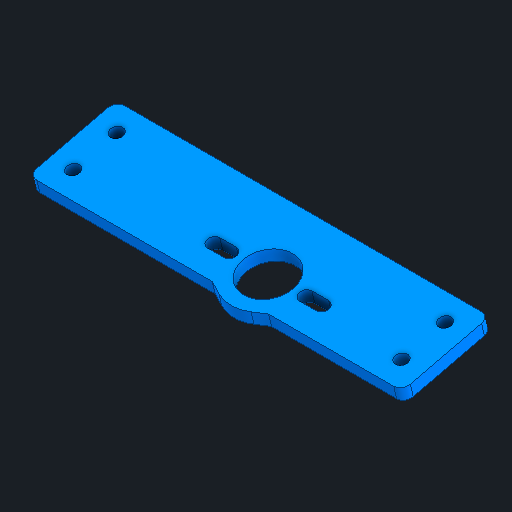
# Autodesk Inventor part: motor_mount_plate
Saved by Autodesk Inventor 2024 (Build 280153000, 153)
## iProperties
Created: 2022-03-30
Part Number: motor_mount_plate
Material: Generic
Document SubType Name: Modeling
Designer: kardo
Density: 1 g/cm^3
Appearance: Blue Plastic
Mass: 3.74158 g
Surface Area: 43.0769 cm^2
Volume: 3.74158 cm^3
Author: kardo
Autodesk Inventor part; units mm, degrees
ref_plane "YZ Plane" through (0, 0, 0) normal (1, 0, 0) x (0, 1, 0)
ref_plane "XZ Plane" through (0, 0, 0) normal (0, 1, 0) x (-1, 0, 0)
ref_plane "XY Plane" through (0, 0, 0) normal (0, 0, 1) x (1, 0, 0)
derived "stencil_frame.ipt"
sketch "sk_cowl_joint_locations" plane through (54.6, 0, 0) normal (1, 0, 0) x (0, 1, 0)
  line L0 (-345, 16.32) -> (-262.2001, 18.586) construction
  arc A0 (-262.2001, 18.586) -> (-241.5001, 19.2432) centre (-326.8578, 2381.2399) ccw construction
  line L1 (-241.5001, 19.2432) -> (11.22, 28.376) construction
  arc A1 (36.465, 28.832) -> (11.22, 28.376) centre (36.465, -670.197) ccw construction
  line L2 (36.465, 28.832) -> (112.2, 28.832) construction
  line L3 (94.8, 29.632) -> (36.465, 29.632) construction
  arc A2 (36.465, 29.632) -> (11.1911, 29.1755) centre (36.465, -670.197) ccw construction
  line L4 (11.1911, 29.1755) -> (-241.529, 20.0427) construction
  arc A3 (-262.222, 19.3857) -> (-241.529, 20.0427) centre (-326.8578, 2381.2399) ccw construction
  line L5 (-262.222, 19.3857) -> (-345, 17.1203) construction
  line L6 (-230.0001, 3089.1136) -> (-230.0001, -1866.0023) construction
  line L7 (-114.9999, 3089.1136) -> (-114.9999, -1866.0023) construction
  line L8 (-345, 3089.1136) -> (-345, -1866.0023) construction
  line L9 (0, 3089.1136) -> (0, -1866.0023) construction
  line L10 (-230.0001, 44.8681) -> (-230.0001, 20.4593) construction
  line L11 (-114.9999, 49.7658) -> (-114.9999, 24.6152) construction
  line L12 (-345, 17.1203) -> (-345, 17.1203)
  line L13 (-345, 17.1203) -> (-345, 36.7228) construction
  line L14 (-850.7464, 3011.9134) -> (325.2296, -1886.3794) construction
  line L15 (-344.7454, 36.7228) -> (-345, 39.712) construction
  line L16 (0, 51.4) -> (0, 28.7711) construction
  line L17 (-144.5331, 44.6212) -> (-139.5174, 23.7292) construction
  line L18 (-134.9371, 30.3529) -> (-140.7713, 28.9522) construction
  line L19 (-137.4449, 40.7989) -> (-143.2792, 39.3982) construction
  line L20 (-144.5331, 44.6212) -> (-138.6989, 46.0219) construction
  line L21 (-139.5174, 23.7292) -> (-133.6831, 25.1299) construction
  line L22 (-138.6989, 46.0219) -> (-138.9044, 52.0184) construction
  spline S0 degree 2 poles (-345, 39.712) (-172.656, 54.3934) (0, 54.4) knots 0 0 0 1 1 1
  spline S1 degree 3 poles (0, 54.4) (37.026, 54.4) (80.784, 47.9917) (112.2, 37.536) knots 1 1 1 1 2 2 2 2
  spline S2 degree 3 poles (111.2526, 34.6895) (106.0906, 36.4075) (96.4401, 39.2282) (84.5011, 42.0313) (75.2591, 43.9395) (68.9709, 45.1125) (60.9945, 46.449) (54.5373, 47.4124) (46.413, 48.4791) (39.8882, 49.2203) (31.7426, 50.0013) (25.2514, 50.5076) (17.2112, 50.9875) (9.2661, 51.3118) (3.0567, 51.4) (0, 51.4) knots 1 1 1 1 1.166667 1.291667 1.333333 1.416667 1.458333 1.541667 1.583333 1.666667 1.708333 1.791667 1.833333 1.916667 2 2 2 2
  spline S3 degree 3 poles (0, 51.4) (-19.1698, 51.3993) (-52.712, 51.1604) (-91.0357, 50.4121) (-119.7742, 49.6473) (-138.931, 49.0355) (-162.8744, 48.1436) (-182.0269, 47.3282) (-205.9648, 46.1816) (-225.113, 45.1626) (-249.0455, 43.7615) (-268.1894, 42.5387) (-292.1166, 40.883) (-316.041, 39.1) (-335.1777, 37.5379) (-344.7454, 36.7228) knots 0 0 0 0 0.166667 0.291667 0.333333 0.416667 0.458333 0.541666 0.583333 0.666666 0.708333 0.791666 0.833333 0.916666 1 1 1 1
  point P0 (0, 0)
  point P1 (-345, 26.9216)
  point P2 (-230.0001, 32.6637)
  point P3 (-114.9999, 37.1905)
  point P4 (0, 40.0855)
  point P5 (0, 40.0855)
ref_plane "plane_motor_mount" through (0, -127.65, 0) normal (0, 0.9723699, 0.2334454) x (-1, 0, 0)
ref_plane "plane_symmetry" through (0, 0, 0) normal (1, 0, 0) x (0, 1, 0)
sketch "sk_drivetrain_profile" plane through (6, 0, 0) normal (1, 0, 0) x (0, 1, 0)
  line L0 (-529.1844, 0) -> (410.1064, 0) construction
  line L1 (-345, 3089.1136) -> (-345, -1866.0023) construction
  line L2 (0, 3089.1136) -> (0, -1866.0023) construction
  line L3 (-140.3859, 53.0487) -> (-133.8494, 25.8223)
  line L4 (-377, 0) -> (-313.1973, 5.0214)
  line L5 (-137.1176, 39.4355) -> (-233.3061, 16.3427)
  line L6 (-296.4782, 6.3372) -> (-264.4984, 8.8541) construction
  line L7 (-264.4984, 8.8541) -> (-233.3061, 16.3427) construction
  line L8 (-133.8494, 25.8223) -> (-133.8494, 20.8223) construction
  line L9 (-313.1973, 5.0214) -> (-296.4782, 6.3372)
  line L10 (-850.7464, 3011.9134) -> (325.2296, -1886.3794) construction
  line L11 (-233.9547, 19.044) -> (-137.7662, 42.1369) construction
  line L12 (-136.4691, 36.7341) -> (-232.6576, 13.6413) construction
  line L13 (-233.9547, 19.044) -> (-232.6576, 13.6413) construction
  spline S0 degree 2 poles (-296.4782, 6.3372) (-264.4984, 8.8541) (-233.3061, 16.3427) knots 1 1 1 2 2 2
  line L14 (0, 21.3303) -> (-241.5001, 18.9703) construction
  line L15 (-55.7851, 21.5852) -> (-309.9218, 19.1017) construction
  point P0 (0, 0)
  point P1 (-221.5492, 19.1653)
  point P2 (-209.1437, 19.2865)
  point P3 (-205.6699, 20.1205)
derived "parameters_frame.ipt"
sketch "sk_base" plane through (0, -127.65, 0) normal (0, 0.9723699, 0.2334454) x (-1, 0, 0)
  line L0 (0, -1324.4284) -> (0, 2990.003) projected
  line L1 (-44.6, 47.3296) -> (-44.6, 25.8439)
  line L2 (-44.6, 25.8439) -> (0, 25.8439)
  line L3 (-44.6, 47.3296) -> (0, 47.3296)
  point P0 (0, -29.7993)
  point P1 (-54.6, 47.3296)
  point P2 (-54.6, 25.8439)
  dimension "d1" = 10
  constraints: 6 end point, 4 point on line, 2 perpendicular, 1 parallel
  measures "d1" distance from line of point (-54.6, 47.33) L1
extrude "base" add sketch "sk_base" against normal blind 3
sketch "sk_drill_joint" plane through (0, -127.65, 0) normal (0, 0.9723699, 0.2334454) x (-1, 0, 0)
  line L0 (-44.6, 47.3296) -> (-44.6, 25.8439) construction
  line L1 (-44.6, 47.3296) -> (0, 47.3296) construction
  line L2 (-44.6, 25.8439) -> (0, 25.8439) construction
  circle A0 centre (-39.2, 31.2439) radius 1.5
  circle A1 centre (-39.2, 41.9296) radius 1.5
  line L3 (-39.2, 41.9296) -> (-39.2, 47.3296) construction
  line L4 (-39.2, 41.9296) -> (-39.2, 31.2439) construction
  line L5 (-39.2, 31.2439) -> (-39.2, 25.8439) construction
  line L6 (-39.2, 41.9296) -> (-44.6, 41.9296) construction
  line L7 (-39.2, 31.2439) -> (-44.6, 31.2439) construction
  point P0 (0, -29.7993)
  dimension "d3" = 3
  dimension "d4" = 5.4
  constraints: 10 end point, 4 perpendicular, 4 point on line, 2 centre point, 2 collinear, 1 coincident, 1 equal radius, 1 parallel
  measures "d3" diameter of A1
  measures "d4" distance between parallel lines of L0 L4
extrude "drill_joint" cut sketch "sk_drill_joint" along normal through all both and the other way through all
mirror "mirror" about plane through (0, 0, 0) normal (1, 0, 0)
sketch "sk_expand_motor" plane through (0, -127.65, 0) normal (0, 0.9723699, 0.2334454) x (-1, 0, 0)
  line L0 (-6, 54.5561) -> (-6, 26.5561) construction
  line L1 (-9.8571, 48.6876) -> (-21.2857, 43.2666)
  arc A0 (-21.2857, 43.2666) -> (-21.2857, 37.8455) centre (-20, 40.5561) ccw
  line L2 (-21.2857, 37.8455) -> (-9.8571, 32.4245)
  arc A1 (-9.8571, 32.4245) -> (-2.1429, 32.4245) centre (-6, 40.5561) ccw
  line L3 (-2.1429, 32.4245) -> (9.2857, 37.8455)
  arc A2 (9.2857, 37.8455) -> (9.2857, 43.2666) centre (8, 40.5561) ccw
  line L4 (9.2857, 43.2666) -> (-2.1429, 48.6876)
  arc A3 (-2.1429, 48.6876) -> (-9.8571, 48.6876) centre (-6, 40.5561) ccw
  line L5 (-20, 40.5561) -> (8, 40.5561) construction
  point P0 (0, -29.7993)
  dimension "d23" = 28
  dimension "d24" = 18
  dimension "d26" = 6
  constraints: 10 end point, 8 point on circle, 8 tangent, 4 centre point, 3 midpoint, 2 coincident, 2 equal radius, 1 perpendicular
  measures "d23" distance of L5.end L5.start
  measures "d24" diameter of A3
  measures "d26" diameter of A2
extrude "expand_motor" add sketch "sk_expand_motor" against normal blind 3
sketch "sk_drill_motor" plane through (0, -127.65, 0) normal (0, 0.9723699, 0.2334454) x (-1, 0, 0)
  circle A0 centre (-6, 40.5561) radius 6
  line L0 (-15, 40.5561) -> (-19, 40.5561) construction
  line L1 (-15, 42.0561) -> (-19, 42.0561)
  line L2 (-19, 39.0561) -> (-15, 39.0561)
  arc A1 (-15, 39.0561) -> (-15, 42.0561) centre (-15, 40.5561) ccw
  arc A2 (-19, 42.0561) -> (-19, 39.0561) centre (-19, 40.5561) ccw
  line L3 (3, 40.5561) -> (7, 40.5561) construction
  line L4 (3, 39.0561) -> (7, 39.0561)
  line L5 (7, 42.0561) -> (3, 42.0561)
  arc A3 (3, 42.0561) -> (3, 39.0561) centre (3, 40.5561) ccw
  arc A4 (7, 39.0561) -> (7, 42.0561) centre (7, 40.5561) ccw
  line L6 (-15, 40.5561) -> (-6, 40.5561) construction
  line L7 (-6, 40.5561) -> (3, 40.5561) construction
  line L8 (-6, 54.5561) -> (-6, 26.5561) construction
  point P0 (0, -29.7993)
  point P1 (-17, 40.5561)
  point P2 (5, 40.5561)
  dimension "d9" = 12
  dimension "d14" = 3
  dimension "d15" = 4
  dimension "d21" = 18
  constraints: 20 end point, 8 point on circle, 8 tangent, 5 centre point, 5 collinear, 2 midpoint, 2 parallel, 1 equal radius, 1 perpendicular
  measures "d9" diameter of A0
  measures "d14" diameter of A2
  measures "d15" distance of L2.start L2.end
  measures "d21" distance of L3.start L0.start
extrude "drill_motor" cut sketch "sk_drill_motor" along normal through all both and the other way through all
fillet "round_corners" radius 2 4 edges at (44.6, -140.1574, 45.6717) (44.6, -135.1417, 24.7797) (-44.6, -140.1574, 45.6717) (-44.6, -135.1417, 24.7797)
derived "parameters_powertrain.ipt"
equation "\"d1\" = cowl_sealing_width + cowl_liner_width"
equation "\"d5\" = bulkhead_thickness"
equation "\"d3\" = drill_motor_mount_diam"
equation "\"d4\" = 1.8 * drill_motor_mount_diam"
equation "\"d27\" = bulkhead_thickness"
equation "\"d18\" = 0.5 * bulkhead_inset"
equation "\"bulkhead_thickness\" = 3"
equation "\"drill_motor_mount_diam\" = 3"
equation "\"bulkhead_inset\" = 4"
equation "\"cowl_sealing_width\" = 5"
equation "\"cowl_liner_width\" = 5"
body "Solid1"
